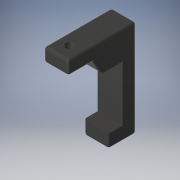
# Autodesk Inventor part: bed_spring_holder_front
Saved by Autodesk Inventor 2018 (Build 220112000, 112)
## iProperties
Created: 2018-05-25
Part Number: bed_spring_holder_front
Material: Plastic, Opaque Black
Document SubType Name: Modeling
Designer: Z. Deniz
Density: 0.952 g/cm^3
Appearance: Smooth - Black
Author: Z. Deniz
Autodesk Inventor part; units mm, degrees
ref_plane "YZ Plane" through (0, 0, 0) normal (1, 0, 0) x (0, 1, 0)
ref_plane "XZ Plane" through (0, 0, 0) normal (0, 1, 0) x (-1, 0, 0)
ref_plane "XY Plane" through (0, 0, 0) normal (0, 0, 1) x (1, 0, 0)
sketch "Sketch1" plane through (0, 0, 0) normal (1, 0, 0) x (0, 1, 0)
  line L0 (0, 0) -> (35, 0)
  line L1 (35, 0) -> (35, 24.5)
  line L2 (35, 24.5) -> (30, 24.5)
  line L3 (30, 24.5) -> (30, 5)
  line L4 (30, 5) -> (5, 5)
  line L5 (5, 5) -> (5, 10)
  line L6 (5, 10) -> (0, 10)
  line L7 (0, 10) -> (0, 0)
  line L8 (25, 5) -> (25, 12.5)
  line L9 (25, 5) -> (32.5, 5) construction
  line L10 (25, 12.5) -> (30, 15.3868)
  dimension "d0" = 35
  dimension "d1" = 24.5
  dimension "d2" = 5
  dimension "d3" = 19.5
  dimension "d9" = 5
  dimension "d10" = 5
  dimension "d23" = 7.5
  dimension "d24" = 90
  dimension "d25" = 120
  dimension "d26" = 5
  constraints: 22 end point, 8 perpendicular, 2 horizontal, 2 point on line, 1 vertical
  measures "d0" distance of L0.start L0.end
  measures "d1" distance of L0.end L1.end
  measures "d2" distance of L1.end L2.end
  measures "d3" distance of L2.end L3.end
  measures "d9" distance of L4.end L5.end
  measures "d10" distance of L5.end L6.end
  measures "d23" distance of L8.start L8.end
  measures "d24" angle of L9 L8
  measures "d25" angle of L8 L10
  measures "d26" distance between parallel lines of L3 L8
extrude "Extrusion1" add sketch "Sketch1" along normal blind 9
sketch "Sketch4" plane through (0, 35, 24.5) normal (0, 1, 0) x (1, 0, 0)
  circle A0 centre (4.5, 5) radius 1.575
  line L0 (0, 0) -> (9, 0) projected
  line L1 (0, 24.5) -> (0, 0) projected
  dimension "d18" = 3.15
  dimension "d19" = 5
  dimension "d20" = 4.5
  constraints: 1 centre point
  measures "d18" diameter of A0
  measures "d19" distance from line of L0 A0.centre
  measures "d20" distance from line of A0.centre L1
extrude "Extrusion3" cut sketch "Sketch4" against normal blind 5
fillet "Fillet1" radius 1 21 edges at (9, 0, 5) (4.5, 0, 10) (0, 0, 5) (4.5, 0, 0) (9, 17.5, 0) (4.5, 30, 15.3868) (4.5, 25, 12.5) (0, 17.5, 0) (9, 35, 12.25) (4.5, 35, 0) (0, 35, 12.25) (4.5, 35, 24.5) (4.5, 30, 24.5) (9, 30, 19.9434) (9, 27.5, 13.9434) (0, 30, 19.9434) (0, 27.5, 13.9434) (9, 32.5, 24.5) (0, 32.5, 24.5) (9, 2.5, 10) (0, 2.5, 10)
body "Solid1"
